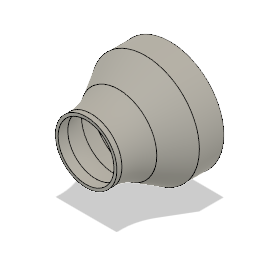
2_5InchFlexHoseTo100mmPVCFitting (Autodesk Fusion 360 design; units mm, degrees)
Autodesk Fusion 360 part; units mm, degrees
sketch "Sketch1" plane through (0, 0, 0) normal (0, 0, 1) x (1, 0, 0)
  circle A0 centre (0, 0) radius 54.75
  circle A1 centre (0, 0) radius 51.75
  dimension "d1" = 109.5
  dimension "d4" = 3
  measures "d1" diameter of A0
  measures "d4" distance of A0 A1
ref_plane "WorkPlane1" through (0, 0, 40) normal (0, 0, 1) x (1, 0, 0)
sketch "Sketch2" plane through (0, 0, 40) normal (0, 0, 1) x (1, 0, 0)
  circle A0 centre (0, 0) radius 31.25
  circle A1 centre (0, 0) radius 28.25
  dimension "d6" = 62.5
  dimension "d8" = 3
  measures "d6" diameter of A0
  measures "d8" distance of A0 A1
extrude "Extrude1" add sketch "Sketch2" along normal blind 20 makes body 1
extrude "Extrude2" add sketch "Sketch1" against normal blind 25 separate body makes body 2
loft "Loft1" add profiles "Sketch1", "Sketch2" section 1 section 2 bodies 1 2
loft "Loft2" cut profiles "Sketch2", "Sketch1" section 1 contours A1 section 2 contours A1 bodies 1
fillet "Fillet1" radius 54.75 1 edges at (-29.1352, -11.3005, 40) on bodies 1
fillet "Fillet2" radius 37.5 2 edges at (-26.3382, 10.2156, 40) (-48.2479, 18.7136, 0) on bodies 1
equation "PVC_OD = 109.5 mm"
equation "wall_thickness = 3 mm"
equation "d4 = wall_thickness"
equation "d6 = Hose_OD"
equation "Hose_OD = 62.50 mm"
equation "d8 = wall_thickness"
